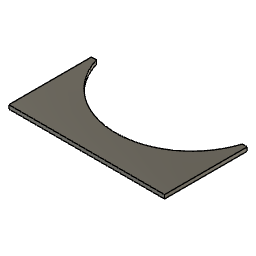
soporte_canal (Autodesk Fusion 360 design; units mm, degrees)
Autodesk Fusion 360 part; units mm, degrees
sketch "Boceto1" plane through (0, 0, 0) normal (0, 0, 1) x (1, 0, 0)
  line L0 (-100.5, 0) -> (-103.5, 0)
  line L1 (101.5, 0) -> (103.5, 0)
  line L2 (103.5, -35) -> (103.5, -140)
  line L3 (103.5, -140) -> (-103.5, -140)
  line L4 (-103.5, -140) -> (-103.5, -35)
  line L5 (-103.5, -35) -> (-100.5, -35)
  line L6 (-100.5, -35) -> (-100.5, -50)
  line L7 (-100.5, -50) -> (-103.5, -50)
  line L8 (-103.5, -50) -> (-103.5, -35)
  line L9 (-103.5, -140) -> (-100.5, -140)
  line L10 (-100.5, -140) -> (-100.5, -125)
  line L11 (-100.5, -125) -> (-103.5, -125)
  line L12 (-103.5, -125) -> (-103.5, -140)
  line L13 (103.5, -140) -> (100.5, -140)
  line L14 (100.5, -140) -> (100.5, -125)
  line L15 (100.5, -125) -> (103.5, -125)
  line L16 (103.5, -125) -> (103.5, -140)
  line L17 (103.5, -35) -> (100.5, -35)
  line L18 (100.5, -35) -> (100.5, -50)
  line L19 (100.5, -50) -> (103.5, -50)
  line L20 (103.5, -50) -> (103.5, -35)
  line L21 (-100.5, -140) -> (-85.5, -140)
  line L22 (-85.5, -140) -> (-85.5, -137)
  line L23 (-85.5, -137) -> (-100.5, -137)
  line L24 (-100.5, -137) -> (-100.5, -140)
  line L25 (100.5, -137) -> (85.5, -137)
  line L26 (85.5, -137) -> (85.5, -140)
  line L27 (85.5, -140) -> (100.5, -140)
  line L28 (100.5, -140) -> (100.5, -137)
  line L29 (103.5, 0) -> (101.5, 0)
  line L30 (-103.5, 0) -> (-101.5, 0)
  arc A0 (-96.9143, -30.1639) -> (96.9143, -30.1639) centre (0, 0) ccw
  line L31 (144.0225, -140) -> (144.0225, -30)
  line L32 (103.5, -30.1639) -> (96.9143, -30.1639)
  line L33 (-96.9143, -30.1639) -> (-103.5, -30.2029)
  line L34 (-103.5, -30.2029) -> (-103.5, -35)
  line L35 (103.5, -30.1639) -> (103.5, -35)
  dimension "d2" = 3
  dimension "d5" = 3
  dimension "d6" = 15
  dimension "d7" = 15
  dimension "d8" = 3
  dimension "d9" = 15
  dimension "d10" = 140
  dimension "d11" = 3
  dimension "d12" = 15
  dimension "d17" = 15
  dimension "d18" = 15
  dimension "d19" = 3
  dimension "d20" = 3
  dimension "d21" = 203
  dimension "d22" = 207
  dimension "d23" = 103.5
  dimension "d24" = 3
  dimension "d25" = 3
  dimension "d26" = 110
  dimension "d27" = 90
  dimension "d28" = 90
  constraint horizontal L0
  constraint horizontal L1
  constraint perpendicular L1 L2
  constraint perpendicular L2 L3
  constraint perpendicular L0 L4
  constraint horizontal L5
  constraint vertical L6
  constraint horizontal L7
  constraint vertical L8
  constraint horizontal L9
  constraint vertical L10
  constraint horizontal L11
  constraint vertical L12
  constraint horizontal L13
  constraint vertical L14
  constraint horizontal L15
  constraint vertical L16
  constraint horizontal L17
  constraint vertical L18
  constraint horizontal L19
  constraint vertical L20
  constraint horizontal L21
  constraint vertical L22
  constraint horizontal L23
  constraint vertical L24
  constraint horizontal L25
  constraint vertical L26
  constraint horizontal L27
  constraint vertical L28
  constraint coincident L14 L25.start
  constraint coincident A0.centre origin
  constraint coincident L0 L30.end
  constraint perpendicular L13 L31
  constraint coincident L2 L32.start
  constraint perpendicular L2 L32
  constraint coincident L4 L33.end
  constraint perpendicular L17 L35
  measures "d2" distance of L0.start L0.end
  measures "d5" distance of L4.end L5.end
  measures "d6" distance of L4.end L7.end
  measures "d7" distance of L3.end L11.end
  measures "d8" distance of L2.end L13.end
  measures "d9" distance of L2.end L15.end
  measures "d10" distance of A0.centre L3
  measures "d11" distance of L2.start L17.end
  measures "d12" distance of L2.start L19.end
  measures "d17" distance of L9.end L21.end
  measures "d18" distance of L25.start L25.end
  measures "d19" distance of L25.end L26.end
  measures "d20" distance of L3 L25
  measures "d21" diameter of A0
  measures "d22" distance of L2 L4
  measures "d23" distance of L4 A0.centre
  measures "d24" distance of L21.end L22.end
  measures "d25" distance of L10.end L11.end
  measures "d26" distance of L31.start L31.end
  measures "d27" distance of L3 L19
  measures "d28" distance of L3 L7
extrude "Extruir3" add sketch "Boceto1" along normal blind 5
extrude "Extruir1" [suppressed]
extrude "Extruir2" [suppressed]
